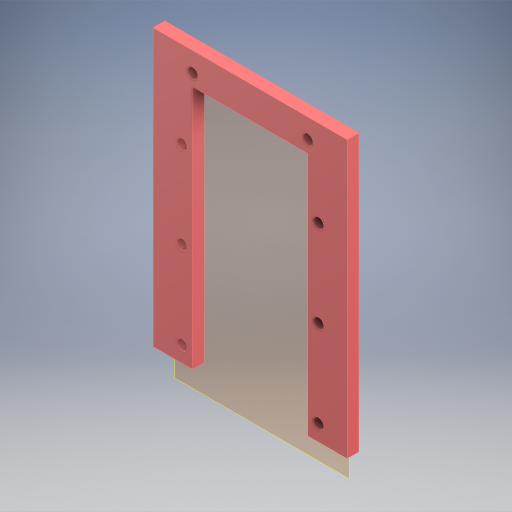
# Autodesk Inventor part: battery_left
Saved by Autodesk Inventor 2024 (Build 280153000, 153)
## iProperties
Created: 2024-09-04
Part Number: battery_left
Material: PMMA 플라스틱
Document SubType Name: Modeling
Designer: msi
Density: 1.188 g/cm^3
Appearance: 매끄러움 - 빨간색
Author: msi
Autodesk Inventor part; units mm, degrees
ref_plane "YZ Plane" through (0, 0, 0) normal (1, 0, 0) x (0, 1, 0)
ref_plane "XZ Plane" through (0, 0, 0) normal (0, 1, 0) x (-1, 0, 0)
ref_plane "XY Plane" through (0, 0, 0) normal (0, 0, 1) x (1, 0, 0)
ref_plane "작업 평면1" through (0, 0, 0) normal (0, 0, 1) x (1, 0, 0)
sketch "스케치1" plane through (0, 0, 0) normal (0, 0, 1) x (1, 0, 0)
  arc A0 (20.1, 4.5766) -> (19.5808, 6.2636) centre (17.1, 4.5766) ccw projected
  line L0 (19.5808, 6.2636) -> (15.5953, 12.1246) projected
  arc A1 (15.5953, 12.1246) -> (13.9414, 13) centre (13.9414, 11) ccw projected
  line L1 (13, 13) -> (13.9414, 13) projected
  arc A2 (14.5, 11.5) -> (13, 13) centre (13, 11.5) ccw projected
  line L2 (14.5, -41.5) -> (14.5, 11.5) projected
  arc A3 (13.5, -42.5) -> (14.5, -41.5) centre (13.5, -41.5) ccw projected
  line L3 (-13.5, -42.5) -> (13.5, -42.5) projected
  arc A4 (-14.5, -41.5) -> (-13.5, -42.5) centre (-13.5, -41.5) ccw projected
  line L4 (-14.5, 11.5) -> (-14.5, -41.5) projected
  arc A5 (-13, 13) -> (-14.5, 11.5) centre (-13, 11.5) ccw projected
  line L5 (-13.9414, 13) -> (-13, 13) projected
  arc A6 (-13.9414, 13) -> (-15.5953, 12.1246) centre (-13.9414, 11) ccw projected
  line L6 (-15.5953, 12.1246) -> (-19.5808, 6.2636) projected
  arc A7 (-19.5808, 6.2636) -> (-20.1, 4.5766) centre (-17.1, 4.5766) ccw projected
  line L7 (-20.1, 4.5766) -> (-20.1, -39.6766) projected
  arc A8 (-20.1, -39.6766) -> (-19.5808, -41.3636) centre (-17.1, -39.6766) ccw projected
  line L8 (-19.5808, -41.3636) -> (-15.8929, -46.7869) projected
  arc A9 (-15.8929, -46.7869) -> (-13.4121, -48.1) centre (-13.4121, -45.1) ccw projected
  line L9 (-13.4121, -48.1) -> (13.4121, -48.1) projected
  arc A10 (13.4121, -48.1) -> (15.8929, -46.7869) centre (13.4121, -45.1) ccw projected
  line L10 (15.8929, -46.7869) -> (19.5808, -41.3636) projected
  arc A11 (19.5808, -41.3636) -> (20.1, -39.6766) centre (17.1, -39.6766) ccw projected
  line L11 (20.1, -39.6766) -> (20.1, 4.5766) projected
  circle A12 centre (-17.3, 4) radius 1.35 projected
  circle A13 centre (-17.3, -18) radius 1.35 projected
  circle A14 centre (-11, -45.3) radius 1.35 projected
  circle A15 centre (17.3, 4) radius 1.35 projected
  circle A16 centre (17.3, -18) radius 1.35 projected
  circle A17 centre (11, -45.3) radius 1.35 projected
  circle A18 centre (-17.3, -40) radius 1.35 projected
  circle A19 centre (17.3, -40) radius 1.35 projected
  arc A20 (-14.6, -41.5) -> (-13.5, -42.6) centre (-13.5, -41.5) ccw
  line L12 (-13.5, -42.6) -> (13.5, -42.6)
  arc A21 (13.5, -42.6) -> (14.6, -41.5) centre (13.5, -41.5) ccw
  arc A22 (13.7746, 12.9) -> (12.2254, 12.9) centre (13, 11.5) ccw
  line L13 (12.2254, 12.9) -> (13.9414, 12.9)
  arc A23 (14.6, 12.7822) -> (13.9414, 12.9) centre (13.9414, 11) ccw
  line L14 (17.6671, -44) -> (15.8102, -46.7307)
  arc A24 (13.4121, -48) -> (15.8102, -46.7307) centre (13.4121, -45.1) ccw
  line L15 (13.4121, -48) -> (-13.4121, -48)
  arc A25 (-15.8102, -46.7307) -> (-13.4121, -48) centre (-13.4121, -45.1) ccw
  line L16 (-15.8102, -46.7307) -> (-17.6671, -44)
  arc A26 (-13.9414, 12.9) -> (-14.6, 12.7822) centre (-13.9414, 11) ccw
  line L17 (-13.9414, 12.9) -> (-12.2254, 12.9)
  arc A27 (-12.2254, 12.9) -> (-14.6, 11.5) centre (-13, 11.5) ccw
  line L18 (-14.6, 11.5) -> (-14.6, -41.5)
  line L19 (13, 13) -> (-13, 13)
  line L20 (-14.6, -44) -> (-24.6, -44)
  line L21 (-24.6, -44) -> (-24.6, 18)
  line L22 (-14.6, 18) -> (-14.6, -44)
  line L23 (-14.6, 18) -> (14.6, 18)
  line L24 (14.6, 19.65) -> (14.6, 21)
  line L25 (-24.6, 21) -> (-24.6, 18)
  line L26 (14.6, 21) -> (15.95, 21)
  line L27 (24.6, 21) -> (24.6, -44)
  line L28 (24.6, -44) -> (14.6, -44)
  line L29 (24.6, 21) -> (24.6, 26)
  line L30 (24.6, 26) -> (-24.6, 26)
  line L31 (-24.6, 26) -> (-24.6, 21)
  circle A28 centre (-14.6, 21) radius 1.35
  circle A29 centre (14.6, 21) radius 1.35
  line L32 (-20.1, 21) -> (-20, 21)
  line L33 (13.25, 21) -> (15.95, 21)
  line L34 (14.6, 21) -> (13.25, 21)
  line L35 (-13.25, 21) -> (-15.95, 21)
  line L36 (14.6, 19.65) -> (14.6, 21)
  circle A30 centre (-17.3, 4) radius 1.35
  circle A31 centre (-17.3, -18) radius 1.35
  circle A32 centre (-17.3, -40) radius 1.35
  circle A33 centre (17.3, -40) radius 1.35
  circle A34 centre (17.3, -18) radius 1.35
  circle A35 centre (17.3, 4) radius 1.35
  line L37 (14.6, -44) -> (14.6, -41.5)
  line L38 (14.6, 12.7822) -> (14.6, 18)
  line L39 (14.6, -41.5) -> (14.6, 12.7822)
  point P0 (0, 0)
  point P1 (-14.6, 11.5)
  point P2 (17.788, -44)
  point P3 (-17.788, -44)
  point P4 (-14.6, 12.8885)
  dimension "d0" = 0.1
  dimension "d3" = 10
  dimension "d4" = 62
  dimension "d5" = 3
  dimension "d6" = 10
  dimension "d7" = 5
  dimension "d8" = 2.7
  dimension "d9" = 2.7
  dimension "d10" = 2.7
  dimension "d11" = 2.7
  dimension "d12" = 2.7
  dimension "d13" = 2.7
  dimension "d14" = 2.7
  dimension "d15" = 2.7
  constraints: 56 end point, 21 point on circle, 16 centre point, 11 parallel, 7 coincident, 7 point on line, 6 horizontal, 5 perpendicular, 1 vertical, 6 other
  measures "d0" distance between parallel lines of L4 L18
  measures "d3" distance of L22.start L21.end
  measures "d4" distance of L20.end L21.end
  measures "d5" distance of L24.end L23.end
  measures "d6" distance of L27.end L28.end
  measures "d7" distance of L29.end L29.start
  measures "d8" diameter of A28
  measures "d9" diameter of A29
  measures "d10" diameter of A30
  measures "d11" diameter of A31
  measures "d12" diameter of A32
  measures "d13" diameter of A33
  measures "d14" diameter of A34
  measures "d15" diameter of A35
extrude "돌출2" add sketch "스케치1" along normal blind 3 contours L11 A11 L10 L28 L37 L39 L38 A1 L0 A0 | A0 L0 A1 L38 L23 L22 A6 L6 A7 L7 A8 L8 L20 L21 L25 L31 L30 L29 L27 L28 L10 A11 L11 | L22 L18 L20 L8 A8 L7 A7 L6 A6
